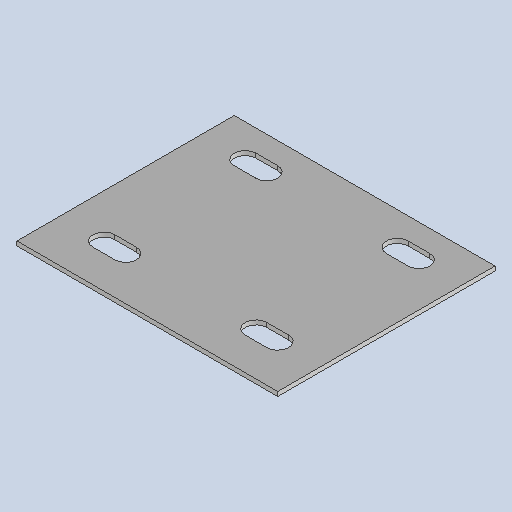
# Autodesk Inventor part: TRM 035 motor pillar 2
Saved by Autodesk Inventor 2025 (Build 290162010, 162A)
## iProperties
Created: 2024-08-07
Part Number: TRM 035 motor pillar 2
Material: AISI 304
Document SubType Name: Sheet Metal
Designer: user
Stock Number: ТРМ 023 лицо успокоитель
Mass: 181.198 g
Surface Area: 238.63 cm^2
Volume: 22.5717 cm^3
Density: 8.02768 g/cm^3
Flat Pattern Width: 12 cm
Flat Pattern Length: 10 cm
Flat Pattern Area: 120 cm^2
Sheet Metal Rule: AISI304 2mm Die16
Sheet Metal Width: 120.000 mm
Sheet Metal Length: 100.000 mm
Sheet Metal Area: 12000.000 mm^2
Appearance: Default
Author: pokla
Autodesk Inventor part; units mm, degrees
ref_plane "YZ Plane" through (0, 0, 0) normal (1, 0, 0) x (0, 1, 0)
ref_plane "XZ Plane" through (0, 0, 0) normal (0, 1, 0) x (-1, 0, 0)
ref_plane "XY Plane" through (0, 0, 0) normal (0, 0, 1) x (1, 0, 0)
sketch "Sketch1" plane through (0, 0, 0) normal (0, 0, 1) x (1, 0, 0)
  line L0 (-60, -50) -> (60, -50)
  line L1 (60, -50) -> (60, 50)
  line L2 (60, 50) -> (-60, 50)
  line L3 (-60, 50) -> (-60, -50)
  line L4 (-60, -50) -> (60, 50) construction
  line L5 (60, -50) -> (-60, 50) construction
  line L6 (-60, 0) -> (60, 0) construction
  line L7 (23.5369, 32.6987) -> (33.5369, 32.6987) construction
  line L8 (23.5369, 27.6987) -> (33.5369, 27.6987)
  line L9 (33.5369, 37.6987) -> (23.5369, 37.6987)
  arc A0 (23.5369, 37.6987) -> (23.5369, 27.6987) centre (23.5369, 32.6987) ccw
  arc A1 (33.5369, 27.6987) -> (33.5369, 37.6987) centre (33.5369, 32.6987) ccw
  point P0 (0, 0)
  point P1 (0, 0)
  point P2 (60, 26.1659)
  point P3 (-14.7466, -50)
  point P4 (28.5369, 32.6987)
  dimension "d0" = 120
  dimension "d1" = 100
  dimension "d17" = 5
  dimension "d18" = 10
  measures "d0" distance of L2.end L1.end
  measures "d1" distance of L1.end L0.end
  measures "d17" radius of A0
  measures "d18" distance of L7.start L7.end
extrude "Plate1" add sketch "Sketch1" along normal blind 2 contours L3 L2 L1 L0 | A0 L9 A1 L8
sketch "Sketch2" plane through (0, 0, 0) normal (0, 0, -1) x (-1, 0, 0)
  line L0 (-40, 30) -> (160, 30) construction
  line L1 (160, 30) -> (160, 10) construction
  line L2 (160, 10) -> (-40, 10) construction
  line L3 (-40, 10) -> (-40, 30) construction
  line L4 (-60, 50) -> (60, 50) projected
  line L5 (-60, -50) -> (-60, 50) projected
  point P0 (0, 0)
  point P1 (-48, 100)
  point P2 (-50, 98)
  point P3 (40, 70)
  point P4 (-60, 26.6315)
  dimension "d6" = 200
  dimension "d9" = 20
  dimension "d10" = 20
  dimension "d11" = 20
  constraints: 4 other
  measures "d6" distance of L0.start L0.end
  measures "d9" distance of L0.end L1.end
  measures "d11" length of L3
mark "Mark1"
sketch "Sketch3" plane through (0, 0, 2) normal (0, 0, 1) x (1, 0, 0)
  line L0 (60, -50) -> (-60, -50) projected
  line L1 (60, 50) -> (60, -50) projected
  line L2 (-60, 50) -> (60, 50) projected
  line L3 (-60, -50) -> (-60, 50) projected
  line L4 (30, 35) -> (40, 35) construction
  line L5 (30, 30) -> (40, 30)
  line L6 (40, 40) -> (30, 40)
  arc A0 (30, 40) -> (30, 30) centre (30, 35) ccw
  arc A1 (40, 30) -> (40, 40) centre (40, 35) ccw
  point P0 (0, 0)
  point P1 (35, 35)
  dimension "d19" = 5
  dimension "d20" = 10
  dimension "d21" = 15
  dimension "d22" = 25
  constraints: 8 end point, 4 point on circle, 4 tangent, 2 centre point, 1 midpoint, 1 parallel
  measures "d19" radius of A0
  measures "d20" distance of L4.start L4.end
  measures "d21" distance between parallel lines of L2 L4
  measures "d22" distance from line of point (35, 35) L1
extrude "Cut1" cut sketch "Sketch3" against normal blind 2 contours A0 L6 A1 L5
pattern_linear "Rectangular Pattern1" count 2 spacing 65 along (0, -1, 0) count 2 spacing 70 along (-1, 0, 0) of "Cut1"
equation "\"d23\" = Thickness"
equation "\"d2\" = Thickness"
equation "\"BendReliefWidth\" = Thickness"
equation "\"BendReliefDepth\" = 0.5 * Thickness"
equation "\"CornerReliefSize\" = 4 * Thickness"
equation "\"MinimumRemnant\" = 2 * Thickness"
equation "\"TransitionRadius\" = BendRadius"
equation "\"JacobiRadiusSize\" = BendRadius"
equation "\"GapSize\" = Thickness"
equation "\"Thickness\" = 2"
equation "\"BendRadius\" = 2.75"
body "Solid1"
